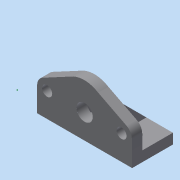
# Autodesk Inventor part: Leadscrew Mount
Saved by Autodesk Inventor 2015 (Build 190159000, 159)
## iProperties
Created: 2016-06-24
Part Number: Leadscrew Mount
Material: Generic
Document SubType Name: Modeling
Designer: Dustin
Density: 1 g/cm^3
Appearance: Default
Author: Dustin
Autodesk Inventor part; units mm, degrees
ref_plane "YZ Plane" through (0, 0, 0) normal (1, 0, 0) x (0, 1, 0)
ref_plane "XZ Plane" through (0, 0, 0) normal (0, 1, 0) x (-1, 0, 0)
ref_plane "XY Plane" through (0, 0, 0) normal (0, 0, 1) x (1, 0, 0)
sketch "Sketch1" plane through (0, 0, 0) normal (0, 0, 1) x (1, 0, 0)
  line L0 (0, 0) -> (50, 0)
  line L1 (50, 0) -> (50, 50)
  line L2 (50, 50) -> (0, 0)
  dimension "d0" = 50
  dimension "d1" = 50
  constraints: 6 end point, 1 horizontal, 1 perpendicular
  measures "d0" distance of L0.end L1.end
  measures "d1" distance of L0.start L0.end
extrude "Extrusion1" add sketch "Sketch1" along normal blind 20
sketch "Sketch2" plane through (0, 0, 20) normal (0, 0, 1) x (1, 0, 0)
  line L0 (50, 50) -> (0, 0) projected
  line L1 (5, 5) -> (45, 5)
  line L2 (45, 5) -> (45, 45)
  line L3 (50, 0) -> (50, 50) projected
  line L4 (0, 0) -> (50, 0) projected
  dimension "d4" = 5
  dimension "d5" = 5
  constraints: 4 end point, 2 point on line, 1 horizontal, 1 perpendicular
  measures "d4" distance between parallel lines of L3 L2
  measures "d5" distance between parallel lines of L4 L1
extrude "Extrusion2" cut sketch "Sketch2" against normal through all contours L2 L1 L0
extrude "Extrusion3" add sketch "Sketch2" against normal blind 5 contours L2 L1 L0
sketch "Sketch3" plane through (0, 0, 0) normal (0, 0, -1) x (-1, 0, 0)
  line L0 (-12.7, 0) -> (-50, 37.3)
  line L1 (-50, 0) -> (-50, 50) projected
  line L2 (-60.6675, 53.6604) -> (-50, 37.3)
  line L3 (-60.6675, 53.6604) -> (-37.4752, 61.571)
  line L4 (-37.4752, 61.571) -> (23.8314, -5.4888)
  line L5 (23.8314, -5.4888) -> (-5.9204, -12.6802)
  line L6 (-5.9204, -12.6802) -> (-12.7, 0)
  point P0 (0, 0)
  dimension "d12" = 12.7
  dimension "d13" = 12.7
  constraints: 12 end point, 1 point on line
  measures "d12" distance of L1.end L0.end
  measures "d13" distance of point (0, 0) L0.start
extrude "Extrusion5" cut sketch "Sketch3" against normal through all
sketch "Sketch4" plane through (0, 0, 15) normal (0, 0, -1) x (-1, 0, 0)
  line L0 (-17.7, 5) -> (-45, 32.3) projected
  line L1 (-45, 5) -> (-45, 32.3) projected
  point P0 (0, 0)
  point P1 (-38, 12)
  dimension "d17" = 7
  dimension "d27" = 7
  measures "d17" horizontal distance of L1.start point (-38, 12)
  measures "d27" distance from line of L1 point (-38, 12)
hole "Hole1" at (38, 12, 15) direction (0, 0, 1) diameter 8 depth 25.4 tip angle 118
sketch "Sketch5" plane through (45, 5, 0) normal (-1, 0, 0) x (0, 0, 1)
  line L0 (0, 0) -> (0, 27.3) projected
  line L1 (20, -5) -> (0, -5) projected
  point P0 (10, 22)
  point P1 (10, 7)
  dimension "d28" = 10
  dimension "d29" = 10
  dimension "d30" = 15
  dimension "d31" = 12
  measures "d28" distance from line of L0 point (10, 7)
  measures "d29" distance from line of L0 point (10, 22)
  measures "d30" distance of point (10, 7) point (10, 22)
  measures "d31" distance from line of L1 point (10, 7)
hole "Hole2" at (45, 27, 10) at (45, 12, 10) direction (1, 0, 0) diameter 5 depth 25.4 tip angle 118
sketch "Sketch6" plane through (45, 5, 15) normal (0, 1, 0) x (1, 0, 0)
  line L0 (-27.3, 15) -> (0, 15) projected
  line L1 (5, 15) -> (5, -5) projected
  point P0 (-45, 15)
  point P1 (-7, 5)
  point P2 (-22, 5)
  dimension "d39" = 15
  dimension "d40" = 10
  dimension "d41" = 10
  dimension "d42" = 12
  measures "d39" distance of point (-7, 5) point (-22, 5)
  measures "d40" distance from line of L0 point (-7, 5)
  measures "d41" distance from line of L0 point (-22, 5)
  measures "d42" distance from line of L1 point (-7, 5)
hole "Hole3" at (38, 5, 10) at (23, 5, 10) direction (0, -1, 0) diameter 5 depth 25.4 tip angle 118
sketch "Sketch7" plane through (0, 0, 0) normal (0, 0, -1) x (-1, 0, 0)
  line L0 (-17.7, 5) -> (-17.7, 0)
  line L1 (-12.7, 0) -> (-50, 0) projected
  line L2 (-17.7, 0) -> (-12.7, 0)
  line L3 (-12.7, 0) -> (-17.7, 5)
  line L4 (-12.7, 0) -> (-17.7, 5) projected
  line L5 (-45, 32.3) -> (-50, 32.3)
  line L6 (-50, 0) -> (-50, 37.3) projected
  line L7 (-50, 32.3) -> (-50, 37.3)
  line L8 (-50, 37.3) -> (-45, 32.3)
  line L9 (-45, 32.3) -> (-50, 37.3) projected
  point P0 (0, 0)
  constraints: 12 end point, 3 collinear, 2 horizontal, 2 point on line, 1 vertical
extrude "Extrusion6" cut sketch "Sketch7" against normal blind 25.4
sketch "Sketch8" plane through (0, 0, 0) normal (0, 0, -1) x (-1, 0, 0)
  line L0 (-17.7, 0) -> (-50, 0) projected
  line L1 (-38, 0) -> (-60.6544, 0)
  line L2 (-60.6544, 0) -> (-60.6544, 37.4521)
  line L3 (-60.6544, 37.4521) -> (-38, 37.4521)
  line L4 (-38, 37.4521) -> (-38, 0)
  circle A0 centre (-38, 12) radius 4 projected
  point P0 (0, 0)
  dimension "d52" = 0
  constraints: 8 end point, 2 parallel, 1 horizontal, 1 perpendicular, 1 point on line
  measures "d52" distance from line of A0.centre L4
extrude "Extrusion7" cut sketch "Sketch8" against normal through all contours L0 L1 L2 L3 L4 A0 | A0 L4 picked at (-39.3236, 12.1607)
mirror "Mirror1" about plane through (38, 37.4521, 0) normal (1, 0, 0)
sketch "Sketch9" plane through (0, 0, 15) normal (0, 0, -1) x (-1, 0, 0)
  point P0 (0, 0)
fillet "Fillet1" radius 8 1 edges at (38, 25.3, 17.5)
sketch "Sketch10" plane through (0, 0, 20) normal (0, 0, 1) x (1, 0, 0)
  arc A0 (9.2418, 17.7) -> (17.7, 5) centre (17.0156, 13.7108) ccw
  arc A1 (58.3, 5) -> (66.7582, 17.7) centre (58.9844, 13.7108) ccw
  arc A2 (66.7582, 17.7) -> (9.2418, 17.7) centre (38, 2.9422) ccw
  line L0 (17.7, 5) -> (32.3431, 19.6431)
  line L1 (32.3431, 19.6431) -> (17.7, 5) projected
  line L2 (58.3, 5) -> (43.6569, 19.6431)
  arc A3 (43.6569, 19.6431) -> (32.3431, 19.6431) centre (38, 13.9863) ccw projected
  line L3 (58.3, 5) -> (43.6569, 19.6431) projected
  arc A4 (43.6569, 19.6431) -> (32.3431, 19.6431) centre (38, 13.9863) ccw
  point P0 (0, 0)
  dimension "d56" = 8.7376
  dimension "d57" = 8.4582
  dimension "d58" = 12.7
  dimension "d59" = 12.7
  dimension "d60" = 8.4582
  dimension "d61" = 0
  constraints: 9 point on circle, 5 tangent, 4 centre point, 4 end point, 2 collinear
  measures "d56" radius of A0
  measures "d57" horizontal distance of L0.start A0.start
  measures "d58" vertical distance of L0.start A0.start
  measures "d59" vertical distance of A1.end L2.start
  measures "d60" horizontal distance of L2.start A1.end
  measures "d61" vertical distance of A1.centre A0.centre
extrude "Extrusion8" add sketch "Sketch10" against normal up to surface (5 mm away)
sketch "Sketch11" plane through (0, 0, 20) normal (0, 0, 1) x (1, 0, 0)
  line L0 (7.4707, 29.1069) -> (71.5137, 29.1069) construction
  line L1 (71.5137, 29.1069) -> (71.5137, -5.7052) construction
  line L2 (71.5137, -5.7052) -> (7.4707, -5.7052) construction
  line L3 (7.4707, -5.7052) -> (7.4707, 29.1069) construction
  point P0 (0, 0)
  constraints: 2 other
sketch "Sketch12" plane through (0, 0, 20) normal (0, 0, 1) x (1, 0, 0)
  arc A0 (17.7, 16.5588) -> (17.7, 7.2332) centre (19.8547, 11.896) ccw
  line L0 (17.7, 16.5588) -> (31.0503, 23.6999)
  arc A1 (44.6361, 23.6999) -> (31.0503, 23.6999) centre (37.8432, 12.753) ccw
  line L1 (58.3, 5) -> (63.7675, 1.1638)
  line L2 (63.7675, 1.1638) -> (73.9162, 6.1166)
  line L3 (73.9162, 6.1166) -> (79.7366, 33.6983)
  line L4 (79.7366, 33.6983) -> (40.092, 40.6944)
  line L5 (40.092, 40.6944) -> (0, 39.3618)
  line L6 (0, 39.3618) -> (-15.8768, 5)
  arc A2 (-15.8768, 5) -> (-14.2095, 1.1638) centre (-13.3336, 3.8249) ccw
  line L7 (-14.2095, 1.1638) -> (10.6084, -22.6037)
  line L8 (10.6084, -22.6037) -> (17.7, 5)
  line L9 (17.7, 7.2332) -> (17.7, 5)
  line L10 (58.3, 7.7519) -> (58.3, 5)
  line L11 (44.6361, 23.6999) -> (58.3, 16.7272)
  arc A3 (58.3, 7.7519) -> (58.3, 16.7272) centre (56.2845, 12.2396) ccw
  point P0 (0, 0)
  constraints: 24 end point, 8 point on circle, 4 centre point, 2 vertical, 1 tangent
extrude "Extrusion9" cut sketch "Sketch12" against normal through all
sketch "Sketch13" plane through (0, 0, 20) normal (0, 0, 1) x (1, 0, 0)
  circle A0 centre (19.6322, 11.9106) radius 2.4728
  circle A1 centre (56.125, 12.2133) radius 2.4552
  point P0 (0, 0)
  constraints: 2 centre point
extrude "Extrusion10" cut sketch "Sketch13" against normal blind 25.4
sketch "Sketch14" plane through (17.7, 5, 15) normal (0, 1, 0) x (1, 0, 0)
  line L0 (26.9361, 0) -> (13.3503, 0) projected
  line L1 (10, 15) -> (15, 15)
  line L2 (15, 15) -> (15, 0)
  line L3 (15, 0) -> (10, 0)
  line L4 (10, 0) -> (10, 15)
  line L5 (40.6, 15) -> (0, 15) projected
  line L6 (25.6, 15) -> (30.6, 15)
  line L7 (30.6, 15) -> (30.6, 0)
  line L8 (30.6, 0) -> (25.6, 0)
  line L9 (25.6, 0) -> (25.6, 15)
  line L10 (40.6, 15) -> (40.6, 0) projected
  line L11 (0, 15) -> (0, 0) projected
  point P0 (-17.7, 15)
  dimension "d83" = 10
  dimension "d84" = 5
  dimension "d85" = 10
  dimension "d86" = 5
  constraints: 16 end point, 4 parallel, 3 point on line, 2 horizontal, 2 perpendicular
  measures "d83" distance between parallel lines of L10 L7
  measures "d84" distance between parallel lines of L7 L9
  measures "d85" distance between parallel lines of L11 L4
  measures "d86" distance between parallel lines of L2 L4
extrude "Extrusion11" add sketch "Sketch14" along normal blind 15 contours L0 L9 L5 L7 L8 | L0 L3 L4 L1 L2
chamfer "Chamfer1" distance 15 angle 45 2 edges at (45.8, 20, 0) (30.2, 20, 0)
sketch "Sketch15" plane through (58.3, 0, 0) normal (1, 0, 0) x (0, 0, -1)
  line L0 (-20, 7.7519) -> (-20, 0) projected
  line L1 (-20, 0) -> (0, 0) projected
  line L2 (0, 0) -> (0, 5) projected
  line L3 (0, 5) -> (-15, 5) projected
  line L4 (-15, 7.7519) -> (-15, 5) projected
  line L5 (-20, 7.7519) -> (-15, 7.7519) projected
  point P0 (0, 0)
extrude "Extrusion12" add sketch "Sketch15" along normal blind 3
sketch "Sketch16" plane through (17.7, 0, 0) normal (-1, 0, 0) x (0, 0, 1)
  line L0 (20, 7.2332) -> (20, 0) projected
  line L1 (20, 7.2332) -> (15, 7.2332) projected
  line L2 (15, 5) -> (15, 7.2332) projected
  line L3 (0, 5) -> (15, 5) projected
  line L4 (0, 0) -> (0, 5) projected
  line L5 (20, 0) -> (0, 0) projected
extrude "Extrusion13" add sketch "Sketch16" along normal blind 3
sketch "Sketch17" plane through (0, 0, 15) normal (0, 0, -1) x (-1, 0, 0)
  line L0 (-14.7, 7.2332) -> (-14.7181, 11.916)
  arc A0 (-17.7, 7.2332) -> (-17.7, 16.5588) centre (-19.8547, 11.896) ccw projected
  line L1 (-14.7181, 11.916) -> (-19.0926, 6.6114)
  line L2 (-19.0926, 6.6114) -> (-14.7, 7.2332)
  line L3 (-61.3, 7.7519) -> (-61.2028, 12.3437)
  arc A1 (-58.3, 16.7272) -> (-58.3, 7.7519) centre (-56.2845, 12.2396) ccw projected
  line L4 (-61.2028, 12.3437) -> (-58.3, 7.7519)
  line L5 (-58.3, 7.7519) -> (-58.6002, 6.2246)
  line L6 (-58.6002, 6.2246) -> (-61.3, 7.7519)
  point P0 (0, 0)
  constraints: 14 end point, 3 point on circle, 2 tangent
extrude "Extrusion14" add sketch "Sketch17" against normal up to surface (5 mm away) contours L2 L1 L0 | L3 A1 L5 L6
body "Solid1"
